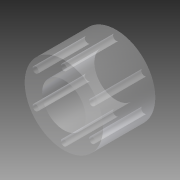
# Autodesk Inventor part: Spacer Between Wheels V2
Saved by Autodesk Inventor 2014 SP1 (Build 180222100, 222)
## iProperties
Created: 2012-01-14
Part Number: Spacer Between Wheels V2
Material: Polycarbonate, Clear
Document SubType Name: Modeling
Designer: actoennies
Density: 1.2 g/cm^3
Mass: 76.7286 g
Surface Area: 172.261 cm^2
Volume: 63.9405 cm^3
Appearance: Polycarbonate - Clear
Author: actoennies
Autodesk Inventor part; units mm, degrees
ref_plane "YZ Plane" through (0, 0, 0) normal (1, 0, 0) x (0, 1, 0)
ref_plane "XZ Plane" through (0, 0, 0) normal (0, 1, 0) x (-1, 0, 0)
ref_plane "XY Plane" through (0, 0, 0) normal (0, 0, 1) x (1, 0, 0)
sketch "Sketch1" plane through (0, 0, 0) normal (0, 0, 1) x (1, 0, 0)
  circle A0 centre (0, 0) radius 15.875
  circle A1 centre (0, 0) radius 23.8125 construction
  circle A2 centre (0, 23.8125) radius 2.2479
  circle A3 centre (-20.6222, 11.9063) radius 2.2479
  circle A4 centre (-20.6222, -11.9062) radius 2.2479
  circle A5 centre (0, -23.8125) radius 2.2479
  circle A6 centre (20.6222, -11.9063) radius 2.2479
  circle A7 centre (20.6222, 11.9062) radius 2.2479
  circle A8 centre (0, 0) radius 28.575
  dimension "d1" = 47.625
  dimension "d0" = 31.75
  dimension "d2" = 4.4958
  dimension "d5" = 360
  dimension "d7" = 57.15
  constraints: 8 centre point, 2 coincident, 1 vertical alignment, 15 other
  measures "d0" diameter of A0
  measures "d2" diameter of A2
  measures "d7" diameter of A8
extrude "Extrusion1" add sketch "Sketch1" along normal blind 38.1
body "Solid1"
